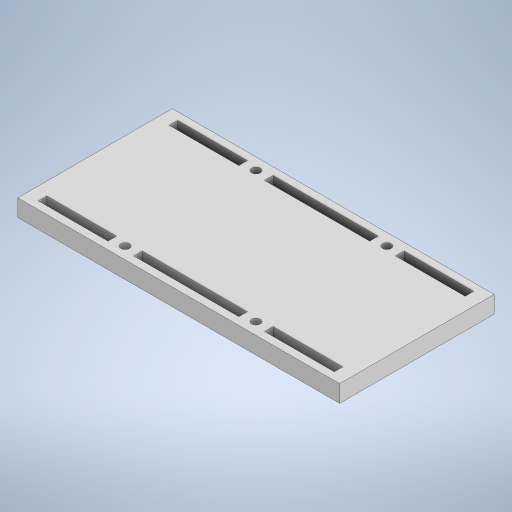
# Autodesk Inventor part: base
Saved by Autodesk Inventor 2024 (Build 280153000, 153)
## iProperties
Created: 2023-05-17
Part Number: base
Material: Generic
Document SubType Name: Modeling
Designer: chris
Density: 1 g/cm^3
Appearance: Default
Author: chris
Autodesk Inventor part; units mm, degrees
ref_plane "YZ Plane" through (0, 0, 0) normal (1, 0, 0) x (0, 1, 0)
ref_plane "XZ Plane" through (0, 0, 0) normal (0, 1, 0) x (-1, 0, 0)
ref_plane "XY Plane" through (0, 0, 0) normal (0, 0, 1) x (1, 0, 0)
sketch "Sketch1" plane through (0, 0, 0) normal (0, 1, 0) x (-1, 0, 0)
  line L0 (0, 0) -> (36, 0)
  line L1 (36, 0) -> (36, -36)
  line L2 (36, -36) -> (0, -36)
  line L3 (0, -36) -> (0, 0)
  line L4 (0, 0) -> (18, 0)
  line L5 (18, 0) -> (18, -18)
  line L6 (18, -18) -> (0, -18)
  line L7 (0, -18) -> (0, 0)
  line L8 (18, -18) -> (33.25, -18)
  line L9 (33.25, -18) -> (33.25, -33.25)
  line L10 (33.25, -33.25) -> (18, -33.25)
  line L11 (18, -33.25) -> (18, -18)
  line L12 (33.25, -33.25) -> (2.75, -33.25)
  line L13 (2.75, -33.25) -> (2.75, -2.75)
  line L14 (2.75, -2.75) -> (33.25, -2.75)
  line L15 (33.25, -2.75) -> (33.25, -33.25)
  circle A0 centre (33.25, -2.75) radius 1
  circle A1 centre (33.25, -33.25) radius 1
  circle A2 centre (2.75, -33.25) radius 1
  circle A3 centre (2.75, -2.75) radius 1
  line L16 (18, -18) -> (55.5, -18)
  line L17 (55.5, -18) -> (55.5, 0)
  line L18 (55.5, 0) -> (18, 0)
  line L19 (18, 0) -> (18, -18)
  line L20 (55.5, 0) -> (-19.5, 0)
  line L21 (-19.5, 0) -> (-19.5, -36)
  line L22 (-19.5, -36) -> (55.5, -36)
  line L23 (55.5, -36) -> (55.5, 0)
  line L24 (-19.5, 0) -> (55.5, 0)
  line L25 (55.5, 0) -> (55.5, 10)
  line L26 (55.5, 10) -> (-19.5, 10)
  line L27 (-19.5, 10) -> (-19.5, 0)
  line L28 (-19.5, -36) -> (55.5, -36)
  line L29 (55.5, -36) -> (55.5, -46)
  line L30 (55.5, -46) -> (-19.5, -46)
  line L31 (-19.5, -46) -> (-19.5, -36)
  dimension "d0" = 36
  dimension "d1" = 36
  dimension "d2" = 18
  dimension "d3" = 18
  dimension "d4" = 15.25
  dimension "d5" = 15.25
  dimension "d6" = 30.5
  dimension "d7" = 30.5
  dimension "d8" = 2
  dimension "d9" = 2
  dimension "d10" = 2
  dimension "d11" = 2
  dimension "d12" = 37.5
  dimension "d13" = 75
  dimension "d16" = 75
  dimension "d17" = 10
  dimension "d18" = 75
  dimension "d19" = 10
  constraints: 64 end point, 16 parallel, 8 horizontal, 8 perpendicular, 4 centre point, 4 coincident
  measures "d0" distance of L1.end L2.end
  measures "d1" distance of L0.end L1.end
  measures "d2" distance of L5.end L6.end
  measures "d3" distance of L4.end L5.end
  measures "d4" distance of L9.end L10.end
  measures "d5" distance of L8.end L9.end
  measures "d6" distance of L13.end L14.end
  measures "d7" distance of L12.end L13.end
  measures "d8" diameter of A0
  measures "d9" diameter of A1
  measures "d10" diameter of A2
  measures "d11" diameter of A3
  measures "d12" distance of L18.end L17.end
  measures "d13" distance of L22.end L21.end
  measures "d16" distance of L26.end L25.end
  measures "d17" distance of L25.end L24.end
  measures "d18" distance of L29.end L30.end
  measures "d19" distance of L28.end L29.end
extrude "Extrusion1" add sketch "Sketch1" along normal blind 4 contours L0 L5 L14 A3 L13 L6 L3 | L3 L22 L21 L20 | L0 L1 L16 L15 A0 L14 L5 | L6 L13 A2 L12 L10 A1 L9 L16 L1 L2 L3 | L18 L17 L16 L1 | L14 A0 L15 L8 L5 | L5 L6 L13 A3 L14 | L6 L11 L12 A2 L13 | L16 L23 L22 L1 | L8 L9 A1 L10 L11
sketch "Sketch2" plane through (0, 4, 0) normal (0, 1, 0) x (1, 0, 0)
  circle A0 centre (-33.25, 2.75) radius 1 projected
  line L0 (-33.25, 3.75) -> (-33.25, 1.75)
  line L1 (-33.25, 3.75) -> (-30.25, 3.75)
  line L2 (-30.25, 3.75) -> (-30.25, 1.75)
  line L3 (-30.25, 1.75) -> (-33.25, 1.75)
  line L4 (-33.25, 1.75) -> (-33.25, 3.75)
  line L5 (-30.25, 1.75) -> (-30.25, 3.75)
  line L6 (-55.5, 0) -> (19.5, 0) projected
  line L7 (19.5, 0) -> (19.5, 36) projected
  line L8 (-55.5, 0) -> (19.5, 0)
  line L9 (19.5, 0) -> (19.5, 18)
  line L10 (19.5, 18) -> (-55.5, 18)
  line L11 (-55.5, 18) -> (-55.5, 0)
  line L12 (-33.25, 3.75) -> (-55.5, 3.75)
  line L13 (-55.5, 3.75) -> (-55.5, 1.75)
  line L14 (-55.5, 1.75) -> (-33.25, 1.75)
  line L15 (-33.25, 1.75) -> (-33.25, 3.75)
  line L16 (-33.25, 3.75) -> (-36.25, 3.75)
  line L17 (-36.25, 3.75) -> (-36.25, 1.75)
  line L18 (-36.25, 1.75) -> (-33.25, 1.75)
  line L19 (-33.25, 1.75) -> (-33.25, 3.75)
  line L20 (-55.5, 3.75) -> (-52.5, 3.75)
  line L21 (-52.5, 3.75) -> (-52.5, 1.75)
  line L22 (-52.5, 1.75) -> (-55.5, 1.75)
  line L23 (-55.5, 1.75) -> (-55.5, 3.75)
  line L24 (-55.5, 36) -> (-55.5, 0) projected
  line L25 (-55.5, 36) -> (-18, 36)
  line L26 (-18, 36) -> (-18, 0)
  line L27 (-18, 0) -> (-55.5, 0)
  line L28 (-55.5, 0) -> (-55.5, 36)
  line L29 (-30.25, 3.75) -> (-18, 3.75)
  line L30 (-18, 3.75) -> (-18, 1.75)
  line L31 (-18, 1.75) -> (-30.25, 1.75)
  line L32 (-30.25, 1.75) -> (-30.25, 3.75)
  circle A1 centre (-33.25, 33.25) radius 1
  line L33 (-33.25, 32.25) -> (-33.25, 34.25)
  line L34 (-33.25, 32.25) -> (-30.25, 32.25)
  line L35 (-30.25, 32.25) -> (-30.25, 34.25)
  line L36 (-30.25, 34.25) -> (-33.25, 34.25)
  line L37 (-33.25, 34.25) -> (-33.25, 32.25)
  line L38 (-30.25, 34.25) -> (-30.25, 32.25)
  line L39 (-33.25, 32.25) -> (-55.5, 32.25)
  line L40 (-55.5, 32.25) -> (-55.5, 34.25)
  line L41 (-55.5, 34.25) -> (-33.25, 34.25)
  line L42 (-33.25, 34.25) -> (-33.25, 32.25)
  line L43 (-33.25, 32.25) -> (-36.25, 32.25)
  line L44 (-36.25, 32.25) -> (-36.25, 34.25)
  line L45 (-36.25, 34.25) -> (-33.25, 34.25)
  line L46 (-33.25, 34.25) -> (-33.25, 32.25)
  line L47 (-55.5, 32.25) -> (-52.5, 32.25)
  line L48 (-52.5, 32.25) -> (-52.5, 34.25)
  line L49 (-52.5, 34.25) -> (-55.5, 34.25)
  line L50 (-55.5, 34.25) -> (-55.5, 32.25)
  line L51 (-30.25, 32.25) -> (-18, 32.25)
  line L52 (-18, 32.25) -> (-18, 34.25)
  line L53 (-18, 34.25) -> (-30.25, 34.25)
  line L54 (-30.25, 34.25) -> (-30.25, 32.25)
  circle A2 centre (-2.75, 2.75) radius 1
  line L55 (-2.75, 3.75) -> (-2.75, 1.75)
  line L56 (-2.75, 3.75) -> (-5.75, 3.75)
  line L57 (-5.75, 3.75) -> (-5.75, 1.75)
  line L58 (-5.75, 1.75) -> (-2.75, 1.75)
  line L59 (-2.75, 1.75) -> (-2.75, 3.75)
  line L60 (-5.75, 1.75) -> (-5.75, 3.75)
  line L61 (19.5, 18) -> (19.5, 0)
  line L62 (-2.75, 3.75) -> (19.5, 3.75)
  line L63 (19.5, 3.75) -> (19.5, 1.75)
  line L64 (19.5, 1.75) -> (-2.75, 1.75)
  line L65 (-2.75, 1.75) -> (-2.75, 3.75)
  line L66 (-2.75, 3.75) -> (0.25, 3.75)
  line L67 (0.25, 3.75) -> (0.25, 1.75)
  line L68 (0.25, 1.75) -> (-2.75, 1.75)
  line L69 (-2.75, 1.75) -> (-2.75, 3.75)
  line L70 (19.5, 3.75) -> (16.5, 3.75)
  line L71 (16.5, 3.75) -> (16.5, 1.75)
  line L72 (16.5, 1.75) -> (19.5, 1.75)
  line L73 (19.5, 1.75) -> (19.5, 3.75)
  line L74 (19.5, 36) -> (19.5, 0)
  line L75 (19.5, 36) -> (-18, 36)
  line L76 (-18, 0) -> (19.5, 0)
  line L77 (19.5, 0) -> (19.5, 36)
  line L78 (-5.75, 3.75) -> (-18, 3.75)
  line L79 (-18, 1.75) -> (-5.75, 1.75)
  line L80 (-5.75, 1.75) -> (-5.75, 3.75)
  circle A3 centre (-2.75, 33.25) radius 1
  line L81 (-2.75, 32.25) -> (-2.75, 34.25)
  line L82 (-2.75, 32.25) -> (19.5, 32.25)
  line L83 (19.5, 34.25) -> (-2.75, 34.25)
  line L84 (16.5, 32.25) -> (16.5, 34.25)
  line L85 (19.5, 32.25) -> (16.5, 32.25)
  line L86 (16.5, 34.25) -> (19.5, 34.25)
  line L87 (19.5, 32.25) -> (19.5, 34.25)
  line L88 (19.5, 34.25) -> (19.5, 32.25)
  line L89 (0.25, 32.25) -> (0.25, 34.25)
  line L90 (-2.75, 32.25) -> (0.25, 32.25)
  line L91 (-2.75, 34.25) -> (-2.75, 32.25)
  line L92 (-2.75, 34.25) -> (-2.75, 32.25)
  line L93 (-2.75, 34.25) -> (-2.75, 32.25)
  line L94 (-2.75, 32.25) -> (-5.75, 32.25)
  line L95 (-5.75, 32.25) -> (-5.75, 34.25)
  line L96 (-5.75, 34.25) -> (-5.75, 32.25)
  line L97 (-5.75, 34.25) -> (-2.75, 34.25)
  line L98 (0.25, 34.25) -> (-2.75, 34.25)
  line L99 (-5.75, 34.25) -> (-5.75, 32.25)
  line L100 (-5.75, 32.25) -> (-18, 32.25)
  line L101 (-18, 34.25) -> (-5.75, 34.25)
  dimension "d20" = 3
  dimension "d24" = 3
  dimension "d25" = 3
  constraints: 198 end point, 59 symmetric about line, 14 parallel, 11 point on line, 8 horizontal, 7 perpendicular, 4 vertical alignment, 2 midpoint, 2 vertical, 7 other
  measures "d20" distance of L2.end L3.end
  measures "d24" distance of L18.end L17.end
  measures "d25" distance of L21.end L22.end
extrude "Extrusion2" cut sketch "Sketch2" against normal up to surface (4 mm away) contours L29 L26 L31 L2 | L17 L14 L21 L12 | L78 L57 L79 L26 | L51 L35 L53 L26 | L26 L101 L95 L100 | L62 L71 L64 L67 | L82 L89 L83 L84 | L48 L41 L44 L39
body "Solid1"
